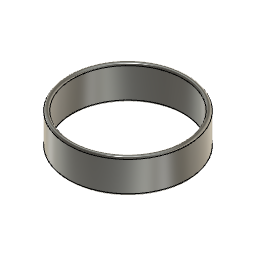
ring (Autodesk Fusion 360 design; units mm, degrees)
Autodesk Fusion 360 part; units mm, degrees
sketch "Sketch1" plane through (0, 0, 0) normal (0, 0, 1) x (1, 0, 0)
  circle A0 centre (0, 0) radius 7
  dimension "d1" = 14
  constraint coincident A0.centre origin
  measures "d1" diameter of A0
extrude "Extrude1" add sketch "Sketch1" along normal blind 4
hole "Hole1" at (0, 0, 4) direction (0, 0, -1) diameter 13 depth 4 tip angle 118
fillet "Fillet1" radius 0.25 2 edges at (-6.0601, 2.3505, 4) (-6.5263, -2.5313, 4)
fillet "Fillet2" radius 0.25 2 edges at (-6.5263, -2.5313, 0) (-6.0601, -2.3505, 0)
